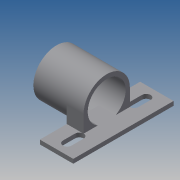
# Autodesk Inventor part: Bearing mount
Saved by Autodesk Inventor 2014 SP1 (Build 180222100, 222)
## iProperties
Created: 2014-02-01
Part Number: Bearing mount
Material: Generic
Document SubType Name: Modeling
Designer: Pradhan Alexander
Density: 1 g/cm^3
Appearance: Default
Author: Pradhan Alexander
Autodesk Inventor part; units mm, degrees
ref_plane "YZ Plane" through (0, 0, 0) normal (1, 0, 0) x (0, 1, 0)
ref_plane "XZ Plane" through (0, 0, 0) normal (0, 1, 0) x (-1, 0, 0)
sketch "Sketch1" plane through (0, 0, 0) normal (0, 1, 0) x (-1, 0, 0)
  line L0 (-3.4844, 10.1285) -> (-28.8844, 10.1285)
  line L1 (-28.8844, 10.1285) -> (-28.8844, -66.0715)
  line L2 (-28.8844, -66.0715) -> (-3.4844, -66.0715)
  line L3 (-3.4844, -66.0715) -> (-3.4844, 10.1285)
  dimension "d0" = 25.4
  dimension "d1" = 76.2
  constraints: 8 end point, 2 parallel, 1 horizontal, 1 perpendicular
  measures "d0" distance of L0.start L0.end
  measures "d1" distance of L2.end L0.start
extrude "Extrusion1" add sketch "Sketch1" against normal blind 3.175
sketch "Sketch7" plane through (3.4844, 0, -66.0715) normal (-1, 0, 0) x (0, 0, 1)
  line L0 (76.2, -3.175) -> (0, -3.175) projected
  circle A0 centre (38.1, 12.7254) radius 6.35
  circle A1 centre (38.1, 12.7254) radius 14.4272
  arc A2 (45.6508, -3.175) -> (30.5492, -3.175) centre (38.1, 12.7254) ccw
  point P0 (38.1, -3.175)
  dimension "d24" = 15.9004
  dimension "d25" = 12.7
  dimension "d26" = 28.8544
  dimension "d57" = 3.175
  constraints: 3 centre point, 2 coincident, 2 point on circle, 2 point on line, 1 midpoint, 1 vertical alignment
  measures "d24" distance from line of L0 A0.centre
  measures "d25" diameter of A0
  measures "d26" diameter of A1
  measures "d57" radial gap between concentric circles of A1 A2
extrude "Extrusion7" add sketch "Sketch7" along normal mid plane 25.4 contours L0 A2
sketch "Sketch8" plane through (16.1844, 0, -66.0715) normal (1, 0, 0) x (0, 0, -1)
  line L0 (-25.9385, 0) -> (-31.3023, 0) projected
  arc A0 (-25.9385, 0) -> (-50.2615, 0) centre (-38.1, 12.7254) ccw projected
  arc A1 (-30.5492, -3.175) -> (-45.6508, -3.175) centre (-38.1, 12.7254) ccw projected
  line L1 (-55.7022, 12.7254) -> (-55.7022, 0)
  line L2 (-50.2615, 0) -> (-76.2, 0) projected
  line L3 (-20.4978, 12.7254) -> (-20.4978, 0)
  line L4 (-76.2, 0) -> (0, 0) projected
  constraints: 4 end point, 4 point on circle, 4 tangent, 2 point on line, 1 parallel, 1 perpendicular
extrude "Extrusion8" add sketch "Sketch8" against normal blind 12.7 contours A0 L3 L4 | L2 L1 A0
sketch "Sketch10" plane through (0, 0, 0) normal (0, 1, 0) x (1, 0, 0)
  arc A0 (12.8824, -2.064) -> (19.4864, -2.064) centre (16.1844, -2.064) ccw
  arc A1 (19.4864, 7.207) -> (12.8824, 7.207) centre (16.1844, 7.207) ccw
  line L0 (12.8824, 7.207) -> (12.8824, -2.064)
  line L1 (19.4864, 7.207) -> (19.4864, -2.064)
  line L2 (19.4864, 2.5715) -> (20.5922, 2.5715)
  line L3 (29.0114, 27.9715) -> (23.9538, 27.9715)
  line L4 (16.1844, 10.509) -> (16.1844, -5.366)
  line L5 (28.8844, 66.0715) -> (3.4844, 66.0715) projected
  line L6 (28.8844, -10.1285) -> (28.8844, 66.0715) projected
  dimension "d43" = 6.604
  dimension "d44" = 6.604
  dimension "d45" = 25.4
  dimension "d53" = 15.875
  constraints: 10 end point, 6 point on circle, 4 tangent, 2 centre point, 1 midpoint, 1 parallel, 1 perpendicular
  measures "d43" diameter of A1
  measures "d44" diameter of A0
  measures "d45" distance between parallel lines of L3 L2
  measures "d53" distance of L4.start L4.end
extrude "Extrusion10" cut sketch "Sketch10" against normal blind 25.4
sketch "Sketch11" plane through (-9.2156, 0, -66.0715) normal (-1, 0, 0) x (0, 0, 1)
  circle A0 centre (38.1, 12.7254) radius 14.4272 projected
  arc A1 (45.6508, -3.175) -> (30.5492, -3.175) centre (38.1, 12.7254) ccw projected
  line L0 (30.5492, -3.175) -> (45.6508, -3.175) projected
extrude "Extrusion11" add sketch "Sketch11" along normal blind 12.7
ref_plane "Work Plane2" through (3.4844, 0, -27.9715) normal (0, 0, 1) x (1, 0, 0)
mirror "Mirror1" about plane through (3.4844, 0, -27.9715) normal (0, 0, 1) of "Extrusion10"
body "Solid1"
